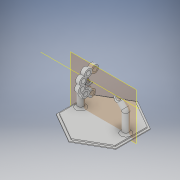
# Autodesk Inventor part: mounter
Saved by Autodesk Inventor 2019 (Build 230136000, 136)
## iProperties
Created: 2018-10-05
Part Number: mounter
Material: Generic
Document SubType Name: Modeling
Designer: HIVE
Density: 1 g/cm^3
Appearance: Default
Author: HIVE
Autodesk Inventor part; units mm, degrees
ref_plane "XZ Plane" through (0, 0, 0) normal (0, 1, 0) x (-1, 0, 0)
sketch "Sketch2" plane through (0, 0, 0) normal (0, 0, 1) x (1, 0, 0)
  line L0 (0, 0) -> (-38.9815, 0)
  line L1 (-46.3001, 0) -> (-38.9815, 0)
  arc A0 (-49.7315, 70) -> (-38.9815, 59.25) centre (-38.9815, 70) ccw
  line L2 (-49.7315, 70) -> (-28.2315, 70)
  arc A1 (-45.7315, 70) -> (-45.0282, 66.9999) centre (-38.9815, 70) ccw
  line L3 (-38.9815, 70) -> (-32.2315, 70) construction
  line L4 (-38.9815, 70) -> (-45.7315, 70) construction
  arc A2 (-38.9815, 59.25) -> (-28.2315, 70) centre (-38.9815, 70) ccw
  line L5 (-38.9815, 0) -> (-31.6629, 0)
  arc A3 (-45.0282, 66.9999) -> (-32.2618, 69.3616) centre (-38.9815, 70) ccw
  arc A4 (-32.2618, 69.3616) -> (-32.2315, 70) centre (-38.9815, 70) ccw
  line L6 (-49.7315, 70) -> (-38.9815, 59.25)
  line L7 (-49.7315, 48.5) -> (-60.4815, 59.25)
  line L8 (-60.4815, 59.25) -> (-49.7315, 70)
  line L9 (-38.9815, 59.25) -> (-49.7315, 48.5)
  line L10 (-49.7315, 48.5) -> (-64.9343, 48.5)
  line L11 (-64.9343, 48.5) -> (-64.9343, 0)
  line L12 (-64.9343, 0) -> (-49.7315, 0)
  line L13 (-49.7315, 0) -> (-49.7315, 48.5)
  arc A5 (-60.4815, 59.25) -> (-64.9343, 48.5) centre (-49.7315, 48.5) ccw
  line L14 (-49.7315, 70) -> (-49.7315, 48.5) construction
  line L15 (-38.9815, 70) -> (-38.9815, 0) construction
  line L16 (-44.3565, 64.625) -> (-55.1065, 53.875)
  line L17 (-57.3329, 48.5) -> (-57.3329, 0)
  arc A6 (-55.1065, 53.875) -> (-57.3329, 48.5) centre (-49.7315, 48.5) ccw
  dimension "d1" = 38.9815
  dimension "d2" = 180
  dimension "d3" = 6.75
  dimension "d4" = 4
  dimension "d5" = 70
  dimension "d32" = 90
  constraints: 37 end point, 14 point on circle, 7 centre point, 4 midpoint, 4 perpendicular, 3 coincident, 3 collinear, 3 horizontal, 2 parallel, 2 point on line, 2 vertical
  measures "d1" distance of L0.start L0.end
  measures "d2" angle of L4 L3
  measures "d3" radius of A1
  measures "d4" radial gap between concentric circles of A0 A1
  measures "d5" distance between parallel lines of L0 L2
revolve "Revolution1" add sketch "Sketch2" angle 55 mid plane about axis through (-49.7315, 70, 0) along (1, 0, 0) contours L6 L16 A0 | L2 A1 A3 A4 A2 L6 | L16 L6 A0
sketch "Sketch3" plane through (0, 0, 0) normal (0, 1, 0) x (-1, 0, 0)
  circle A0 centre (0, 0) radius 87.5
  circle A1 centre (38.9815, 0) radius 7.3186 projected
  line L0 (0, -87.5) -> (-75.7772, -43.75)
  line L1 (-75.7772, -43.75) -> (-75.7772, 43.75)
  line L2 (-75.7772, 43.75) -> (0, 87.5)
  line L3 (0, 87.5) -> (75.7772, 43.75)
  line L4 (75.7772, 43.75) -> (75.7772, -43.75)
  line L5 (75.7772, -43.75) -> (0, -87.5)
  line L6 (-70.7772, -40.8632) -> (0, -81.7265)
  line L7 (0, -81.7265) -> (70.7772, -40.8632)
  line L8 (70.7772, -40.8632) -> (70.7772, 40.8632)
  line L9 (70.7772, 40.8632) -> (0, 81.7265)
  line L10 (0, 81.7265) -> (-70.7772, 40.8632)
  line L11 (-70.7772, 40.8632) -> (-70.7772, -40.8632)
  dimension "d14" = 175
  dimension "d15" = 5
  constraints: 24 end point, 2 coincident, 1 vertical, 1 vertical alignment, 20 other
  measures "d15" distance between parallel lines of L0 L6
extrude "Extrusion3" add sketch "Sketch3" against normal blind 5 contours A1 | L11 L10 L9 L8 L7 L6
extrude "Extrusion4" add sketch "Sketch3" along normal blind 2 from surface at -5 contours L4 L5 L0 L1 L2 L3
sketch "Sketch7" plane through (0, 0, 0) normal (0, 1, 0) x (-1, 0, 0)
  circle A0 centre (57.3329, 0) radius 7.6014
  line L0 (64.9343, 0) -> (49.7315, 0) projected
  point P0 (0, 0)
  point P1 (49.7315, 0)
  constraints: 2 point on circle, 1 centre point, 1 midpoint
sweep "Sweep1" add profiles "Sketch7" path "Sketch2" path curves L17 A6 L16
ref_plane "Work Plane1" through (-38.9815, 70, 0) normal (1, 0, 0) x (0, 1, 0)
sketch "Sketch8" plane through (-38.9815, 70, 0) normal (1, 0, 0) x (0, 1, 0)
  point P0 (-70, 0)
sketch "Sketch10" plane through (-38.9815, 70, 0) normal (1, 0, 0) x (0, 1, 0)
  line L0 (0, 0) -> (-25, 0) construction
  circle A0 centre (-25, 0) radius 5.5
  circle A1 centre (-25, 0) radius 9.5
  circle A2 centre (0, 0) radius 25 construction
  circle A3 centre (-19.2628, 15.9356) radius 9.5
  circle A4 centre (-19.2628, 15.9356) radius 5.5
  circle A5 centre (-4.6845, 24.5572) radius 9.5
  circle A6 centre (-4.6845, 24.5572) radius 5.5
  circle A7 centre (12.0438, 21.9077) radius 9.5
  circle A8 centre (12.0438, 21.9077) radius 5.5
  circle A9 centre (23.2444, 9.2031) radius 9.5
  circle A10 centre (23.2444, 9.2031) radius 5.5
  circle A11 centre (23.7764, -7.7254) radius 9.5
  circle A12 centre (23.7764, -7.7254) radius 5.5
  point P0 (-70, 0)
  dimension "d38" = 11
  dimension "d39" = 4
  dimension "d42" = 198
  dimension "d49" = 25
  constraints: 12 centre point, 2 coincident, 2 end point, 1 horizontal, 1 horizontal alignment, 18 other
  measures "d38" diameter of A0
  measures "d39" radial gap between concentric circles of A0 A1
  measures "d49" distance of L0.start L0.end
extrude "Extrusion7" add sketch "Sketch10" along normal blind 10
extrude "Extrusion8" cut sketch "Sketch10" against normal through all contours A0
extrude "Extrusion9" [suppressed]
fillet "Fillet5" radius 5 1 edges at (-49.7315, 0, 0)
mirror "Mirror4" about plane through (0, 0, 0) normal (1, 0, 0) of "Sweep1", "Revolution1", "Fillet5"
equation "\"d1\" = 0.5 * ballDist"
equation "\"d3\" = 0.5 * ballDiam + clearance"
equation "\"ballDist\" = 77.963"
equation "\"ballDiam\" = 12.7"
equation "\"clearance\" = 0.4"
body "Solid1"
